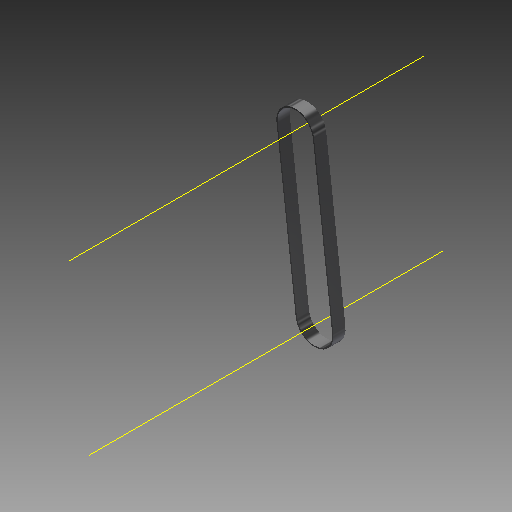
# Autodesk Inventor part: Zahnriemen
Saved by Autodesk Inventor 2017.3 (Build 213256000, 256)
## iProperties
Created: 2018-02-01
Part Number: Zahnriemen
Material: Rubber
Document SubType Name: Modeling
Designer: Dima
Density: 1 g/cm^3
Appearance: Rubber - Black - Version 1.1
CustomPartVersion: 1
Author: Dima
Autodesk Inventor part; units mm, degrees
sketch "Skizzenpfad" plane through (0, 0, 0) normal (0, 0, 1) x (1, 0, 0)
  arc A0 (-5.6516, -125.5142) -> (24.369, -121.8826) centre (9.3587, -123.6984) ccw
  arc A1 (8.4948, 9.3396) -> (-21.5258, 5.7079) centre (-6.5155, 7.5238) ccw
  line L0 (8.4948, 9.3396) -> (24.369, -121.8826)
  line L1 (-5.6516, -125.5142) -> (-21.5258, 5.7079)
  constraints: 4 end point, 4 point on circle, 2 centre point
ref_plane "Querschnittsebene" through (24.369, -121.8826, 0) normal (-0.1201, 0.9928, 0) x (0, 0, 1)
ref_plane "Arbeitsebene2" through (9.3587, -123.6984, 0) normal (-1, 0, 0) x (0, 0, 1)
ref_plane "Arbeitsebene3" through (-6.5155, 7.5238, 0) normal (-0.1037, -0.9946, 0) x (0, 0, 1)
sketch "Querschnitt" plane through (24.369, -121.8826, 0) normal (-0.1201, 0.9928, 0) x (0, 0, 1)
  line L0 (-5, 0.5) -> (5, 0.5)
  line L1 (5, 0.5) -> (5, -0.5)
  line L2 (5, -0.5) -> (-5, -0.5)
  line L3 (-5, -0.5) -> (-5, 0.5)
  line L4 (-5, 0) -> (5, 0) construction
  point P0 (0, 0)
  point P1 (0, 0)
  dimension "d0" = 10
  dimension "d4" = 0.5
  dimension "d5" = 0.5
  constraints: 10 end point, 3 midpoint, 2 parallel, 1 coincident, 1 horizontal, 1 perpendicular, 1 other
  measures "d0" distance between parallel lines of L1 L3
  measures "d4" distance between parallel lines of L2 L4
  measures "d5" distance between parallel lines of L4 L0
sweep "Riemen" add profiles "Querschnitt" path "Skizzenpfad"
equation "\"d0\" = da_B"
equation "\"d4\" = da_a"
equation "\"d5\" = da_a2"
equation "\"da_B\" = 10"
equation "\"da_pb\" = 5"
equation "\"da_L\" = 359.35771"
equation "\"da_a\" = 0.5"
equation "\"da_S\" = 2.65"
equation "\"da_Beta\" = 20deg"
equation "\"da_Ht\" = 1.2"
equation "\"da_H\" = 2.2"
equation "\"da_a2\" = 0.5"
body "Solid1"
